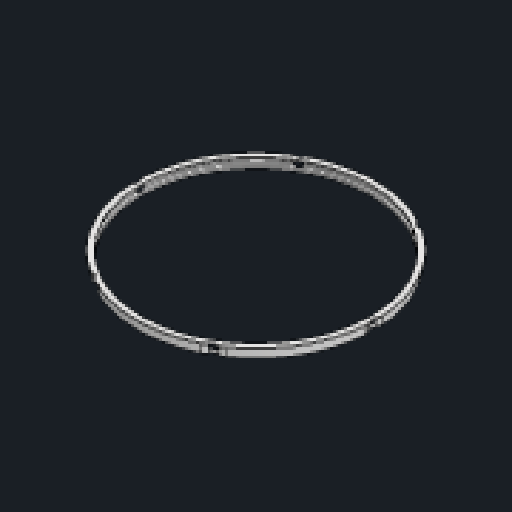
# Autodesk Inventor part: Ring Bearing Track
Saved by Autodesk Inventor 2023.2 (Build 272271030, 271C)
## iProperties
Created: 2024-02-21
Part Number: Ring Bearing Track
Material: Generic
Document SubType Name: Modeling
Designer: robpl
Density: 1 g/cm^3
Appearance: Default
Author: robpl
Autodesk Inventor part; units mm, degrees
ref_plane "YZ Plane" through (0, 0, 0) normal (1, 0, 0) x (0, 1, 0)
ref_plane "XZ Plane" through (0, 0, 0) normal (0, 1, 0) x (-1, 0, 0)
ref_plane "XY Plane" through (0, 0, 0) normal (0, 0, 1) x (1, 0, 0)
sketch "Sketch1" plane through (0, 0, 0) normal (0, 0, 1) x (1, 0, 0)
  line L0 (-67, 0) -> (-70, 0)
  line L1 (-70, 0) -> (-70, 1)
  line L2 (-70, 1) -> (-67, 1)
  line L3 (-67, 1) -> (-67, 0)
  line L4 (-67, 0) -> (-69, 0)
  line L5 (-69, 0) -> (-69, -5)
  line L6 (-69, -5) -> (-67, -5)
  line L7 (-67, -5) -> (-67, 0)
  line L8 (-61.5, -0.5) -> (-67.5, -0.5)
  line L9 (-67.5, -0.5) -> (-67.5, -3)
  line L10 (-67.5, -3) -> (-61.5, -3)
  line L11 (-61.5, -3) -> (-61.5, -0.5)
  line L12 (-67, -3.5) -> (-68, -2.5)
  line L13 (-68, -2.5) -> (-68, -1)
  line L14 (-68, -1) -> (-67, 0)
  line L15 (0, -6.2) -> (0, 2.2) projected
  point P0 (0, 0)
  point P1 (-69, 0)
  point P2 (-67.5, -1.75)
  point P3 (-70, 0.5)
  point P4 (-68, -1.75)
  dimension "d0" = 5
  dimension "d1" = 69
  dimension "d4" = 1
  dimension "d5" = 2.5
  dimension "d6" = 67.5
  dimension "d7" = 67
  dimension "d9" = 3.5
  dimension "d11" = 2
  dimension "d12" = 6
  dimension "d13" = 0.5
  dimension "d27" = 0.5
  dimension "d28" = 1
  constraints: 30 end point, 6 parallel, 6 perpendicular, 5 midpoint, 3 horizontal, 3 point on line
  measures "d0" distance of L6.end L0.start
  measures "d1" distance from line of point (0, 0) L5
  measures "d4" distance of L2.end L0.start
  measures "d5" distance of L10.end L8.start
  measures "d6" distance from line of point (0, 0) L9
  measures "d7" distance from line of point (0, 0) L7
  measures "d9" distance of L12.start L14.end
  measures "d11" distance between parallel lines of L6 L10
  measures "d12" distance of L9.end L10.end
  measures "d13" distance between parallel lines of L9 L3
  measures "d27" distance from line of point (-68, -1.75) L9
  measures "d28" distance between parallel lines of L5 L1
revolve "Revolution1" add sketch "Sketch1" angle 360 about axis through (0, -10, 0) along (0, 1, 0) contours L14 L13 L12 L7 L6 L5 L0 | L0 L1 L2 L3
sketch "Sketch2" plane through (0, 1, 0) normal (0, 1, 0) x (1, 0, 0)
  circle A0 centre (-72.25, 0) radius 2.55
  point P0 (0, 0)
  dimension "d16" = 5.1
  dimension "d17" = 72.25
  constraints: 1 centre point, 1 horizontal alignment
  measures "d16" diameter of A0
  measures "d17" distance of point (0, 0) A0.centre
extrude "Extrusion1" cut sketch "Sketch2" against normal through all
sketch "Sketch3" plane through (0, -5, 0) normal (0, -1, 0) x (0, 0, 1)
  arc A0 (-68.9899, -1.1809) -> (-68.9899, 1.1809) centre (-71.25, 0) ccw projected
  circle A1 centre (-71.25, 0) radius 4
  point P0 (0, 0)
  dimension "d20" = 8
  constraints: 1 centre point, 1 coincident
  measures "d20" diameter of A1
extrude "Extrusion2" [suppressed]
fillet "Fillet1" radius 4 2 edges at (-69.99, 0.5, -1.1811) (-69.99, 0.5, 1.1811)
pattern_circular "Circular Pattern1" [suppressed]
body "Solid1"
